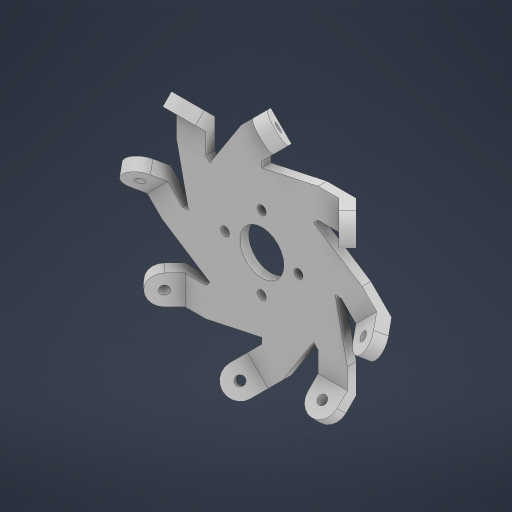
# Autodesk Inventor part: Frame
Saved by Autodesk Inventor 2023 (Build 270158000, 158)
## iProperties
Created: 2023-04-05
Part Number: Frame
Material: Generic
Document SubType Name: Modeling
Designer: vatdu
Density: 1 g/cm^3
Appearance: Default
Author: vatdu
Autodesk Inventor part; units mm, degrees
ref_plane "YZ Plane" through (0, 0, 0) normal (1, 0, 0) x (0, 1, 0)
ref_plane "XZ Plane" through (0, 0, 0) normal (0, 1, 0) x (-1, 0, 0)
sketch "Sketch1" plane through (0, 0, 0) normal (0, 0, 1) x (1, 0, 0)
  circle A0 centre (0, 0) radius 7.5
  circle A1 centre (0, 0) radius 25
  line L0 (0, 0) -> (25, 0) construction
  line L1 (17.6777, 17.6777) -> (19.0919, 19.0919)
  line L2 (19.0919, 19.0919) -> (29.0919, 19.0919)
  line L3 (29.0919, 19.0919) -> (29.0919, 29.0919)
  line L4 (29.0919, 29.0919) -> (19.0919, 29.0919)
  line L5 (19.0919, 29.0919) -> (0, 25)
  line L6 (0, 25) -> (0, 27)
  line L7 (0, 27) -> (7.0711, 34.0711)
  line L8 (7.0711, 34.0711) -> (0, 41.1421)
  line L9 (0, 41.1421) -> (-7.0711, 34.0711)
  line L10 (-7.0711, 34.0711) -> (-17.6777, 17.6777)
  line L11 (-17.6777, 17.6777) -> (-19.0919, 19.0919)
  line L12 (-19.0919, 19.0919) -> (-19.0919, 29.0919)
  line L13 (-19.0919, 29.0919) -> (-29.0919, 29.0919)
  line L14 (-29.0919, 29.0919) -> (-29.0919, 19.0919)
  line L15 (-29.0919, 19.0919) -> (-25, 0)
  line L16 (-25, 0) -> (-27, 0)
  line L17 (-27, 0) -> (-34.0711, 7.0711)
  line L18 (-34.0711, 7.0711) -> (-41.1421, 0)
  line L19 (-41.1421, 0) -> (-34.0711, -7.0711)
  line L20 (-34.0711, -7.0711) -> (-17.6777, -17.6777)
  line L21 (-17.6777, -17.6777) -> (-19.0919, -19.0919)
  line L22 (-19.0919, -19.0919) -> (-29.0919, -19.0919)
  line L23 (-29.0919, -19.0919) -> (-29.0919, -29.0919)
  line L24 (-29.0919, -29.0919) -> (-19.0919, -29.0919)
  line L25 (-19.0919, -29.0919) -> (0, -25)
  line L26 (0, -25) -> (0, -27)
  line L27 (0, -27) -> (-7.0711, -34.0711)
  line L28 (-7.0711, -34.0711) -> (0, -41.1421)
  line L29 (0, -41.1421) -> (7.0711, -34.0711)
  line L30 (7.0711, -34.0711) -> (17.6777, -17.6777)
  line L31 (17.6777, -17.6777) -> (19.0919, -19.0919)
  line L32 (19.0919, -19.0919) -> (19.0919, -29.0919)
  line L33 (19.0919, -29.0919) -> (29.0919, -29.0919)
  line L34 (29.0919, -29.0919) -> (29.0919, -19.0919)
  line L35 (29.0919, -19.0919) -> (25, 0)
  line L36 (25, 0) -> (27, 0)
  line L37 (27, 0) -> (34.0711, -7.0711)
  line L38 (34.0711, -7.0711) -> (41.1421, 0)
  line L39 (41.1421, 0) -> (34.0711, 7.0711)
  line L40 (34.0711, 7.0711) -> (17.6777, 17.6777)
  circle A2 centre (0, 12.5) radius 1.5
  circle A3 centre (12.5, 0) radius 1.5
  circle A4 centre (0, -12.5) radius 1.5
  circle A5 centre (-12.5, 0) radius 1.5
  dimension "d0" = 15
  dimension "d1" = 50
  dimension "d3" = 2
  dimension "d4" = 10
  dimension "d5" = 135
  dimension "d6" = 10
  dimension "d7" = 10
  dimension "d10" = 360
  dimension "d13" = 3
  dimension "d14" = 3
  dimension "d15" = 3
  dimension "d16" = 3
  constraints: 82 end point, 8 point on line, 6 centre point, 2 coincident, 2 horizontal, 2 point on circle, 1 midpoint, 1 perpendicular, 89 other
  measures "d0" diameter of A0
  measures "d1" diameter of A1
  measures "d3" distance of L1.start L1.end
  measures "d4" distance of L1.end L2.end
  measures "d5" angle of L1 L2
  measures "d6" distance of L2.end L3.end
  measures "d7" distance of L3.end L4.end
  measures "d13" diameter of A2
  measures "d14" diameter of A3
  measures "d15" diameter of A4
  measures "d16" diameter of A5
extrude "Extrusion1" add sketch "Sketch1" along normal blind 3
ref_plane "Work Plane1" through (-7.0711, -34.0711, 0) normal (0.5, 0.5, -0.7071068) x (0.7071068, -0.7071068, 0)
sketch "Sketch2" plane through (-7.0711, -34.0711, 0) normal (0.5, 0.5, -0.7071068) x (0.7071068, -0.7071068, 0)
  line L0 (10, 0) -> (10, -7.0711) projected
  line L1 (0, -9.1924) -> (0, -2.1213) projected
  line L2 (10, 0) -> (0, 0)
  line L3 (0, 0) -> (0, -4.2117)
  line L4 (0, -4.2117) -> (10, -4.2117)
  line L5 (10, -4.2117) -> (10, 0)
  point P0 (-19.0919, -20.5711)
  point P1 (0, -2.1213)
  point P2 (10, -4.2117)
  constraints: 8 end point, 2 parallel, 1 horizontal, 1 perpendicular, 1 point on line
extrude "Extrusion2" add sketch "Sketch2" against normal blind 10
fillet "Fillet1" radius 5 2 edges at (-11.0181, -38.0181, 8.5601) (-3.9471, -45.0892, 8.5601)
sketch "Sketch3" plane through (2.0904, -39.0518, 3) normal (0.5, 0.5, 0.7071068) x (0.5, 0.5, -0.7071068)
  line L0 (0, 0) -> (-4.969, 0) projected
  line L1 (0, 10) -> (-4.969, 10) projected
  circle A0 centre (-4.969, 5) radius 1.5
  point P0 (20.602, 29.0919)
  dimension "d23" = 3
  constraints: 1 centre point
  measures "d23" diameter of A0
extrude "Extrusion3" cut sketch "Sketch3" against normal blind 10
pattern_circular "Circular Pattern1" count 8 over 360 about axis through (0, 0, 0) along (0, 0, 1) of "Fillet1", "Extrusion3", "Extrusion2"
body "Solid1"
